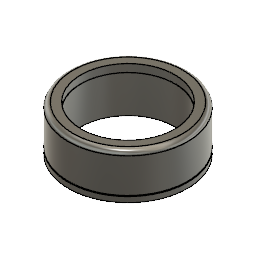
Ikea Lamp adapter v1 (Autodesk Fusion 360 design; units mm, degrees)
Autodesk Fusion 360 part; units mm, degrees
sketch "Sketch1" plane through (0, 0, 0) normal (0, 1, 0) x (1, 0, 0)
  circle A0 centre (0, 0) radius 30.125
  circle A1 centre (0, 0) radius 34.125
  dimension "d1" = 60.25
  dimension "d2" = 4
  constraint coincident A0.centre A1.centre
  measures "d1" diameter of A0
extrude "Extrude1" add sketch "Sketch1" along normal blind 20 makes body 1
sketch "Sketch2" plane through (0, 0, 0) normal (0, -1, 0) x (1, 0, 0)
  circle A0 centre (0, 0) radius 30.125
  circle A1 centre (0, 0) radius 34.125
  circle A2 centre (0, 0) radius 38.125
  circle A3 centre (0, 0) radius 34.325
  dimension "d5" = 4
  dimension "d6" = 0.2
extrude "Extrude2" add sketch "Sketch2" against normal blind 20 separate body contours A2 makes body 2
extrude "Extrude3" add 1 faces at (32.5525, 0, 3.192) along direction (0, -1, 0) blind 4 on bodies 1 bodies 1
extrude "Extrude4" add sketch "Sketch2" along normal blind 4 and the other way blind -0.5 contours A2 | A3 bodies 1
thread "Thread1" "ISO Metric profile 70.0 M70x6 6g" major diameter 69.62 minor diameter 62.7358 pitch 6 angle 60 modelled right hand crest width 0.8424 on face at (33.9554, 6.3333, -3.3978) crest through (34.81, -2, 0) on bodies 1
thread "Thread2" "ISO Metric profile 70.0 M70x6 6H" major diameter 70.6205 minor diameter 63.9048 pitch 6 angle 60 modelled right hand crest width 1.6227 on face at (34.2823, 13.3333, -1.711) crest through (31.9524, 1.5, 0) on bodies 2
sketch "Sketch3" plane through (0, 20, 0) normal (0, 1, 0) x (-1, 0, 0)
  spline S0 degree 3 poles (34.1072, 9.1387) (35.0783, 4.6912) (35.1792, 0.0982) (33.6138, -8.784) (31.9938, -12.9925) (27.2629, -20.4736) (24.2245, -23.6906) (17.1441, -28.7184) (13.189, -30.5063) (6.4794, -32.0634) (3.8971, -32.3471) (-1.2486, -32.2925) (-3.7936, -31.9617) (-6.2718, -31.3308) knots 0 0 0 0 1.365688 1.365688 2.70677 2.70677 4.023239 4.023239 5.315084 5.315084 6.092959 6.092959 6.861523 6.861523 6.861523 6.861523
  arc A0 (-30.2692, 10.2339) -> (-6.2718, -31.3308) centre (0, 0) ccw
  spline S1 degree 3 poles (-30.2692, 10.2339) (-29.1325, 14.2731) (-27.2108, 18.0485) (-21.9881, 24.7265) (-18.7129, 27.545) (-11.2005, 31.8233) (-7.0203, 33.2142) (1.7201, 34.3417) (6.1997, 34.036) (13.1674, 32.1741) (15.7414, 31.1426) (20.619, 28.4789) (22.9016, 26.8497) (24.9679, 24.9683) knots 0 0 0 0 1.25883 1.25883 2.542243 2.542243 3.850232 3.850232 5.182787 5.182787 6.010321 6.010321 6.847146 6.847146 6.847146 6.847146
  arc A1 (34.1072, 9.1387) -> (24.9679, 24.9683) centre (0, 0) ccw
  circle A2 centre (0, 0) radius 38.125
  circle A3 centre (0, 0) radius 38.125
  circle A4 centre (0, 0) radius 30
  dimension "d15" = 60
  constraint concentric A0 A3
  constraint coincident A0.centre A1.centre
  measures "d15" diameter of A4
extrude "Extrude5" add sketch "Sketch3" along normal blind 5 contours S0 A0 S1 A1 | A2 A3 bodies 2
fillet "Fillet1" radius 3 1 edges at (35.545, 25, -13.7866) on bodies 2
